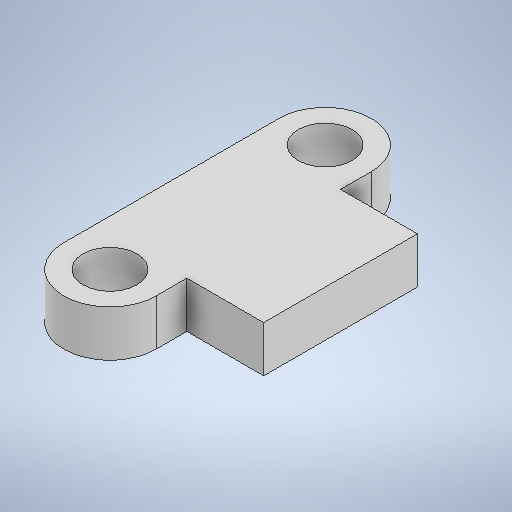
# Autodesk Inventor part: Top Bracket
Saved by Autodesk Inventor 2026.2 (Build 302298010, 298A)
## iProperties
Created: 2026-05-02
Part Number: Top Bracket
Material: Generic
Document SubType Name: Modeling
Designer: piete
Density: 1 g/cm^3
Appearance: Default
Author: piete
Autodesk Inventor part; units mm, degrees
ref_plane "YZ Plane" through (0, 0, 0) normal (1, 0, 0) x (0, 1, 0)
ref_plane "XZ Plane" through (0, 0, 0) normal (0, 1, 0) x (-1, 0, 0)
ref_plane "XY Plane" through (0, 0, 0) normal (0, 0, 1) x (1, 0, 0)
sketch "Sketch1" plane through (0, 0, 0) normal (0, 1, 0) x (-1, 0, 0)
  circle A0 centre (0, 7) radius 1.75
  circle A1 centre (0, -7) radius 1.75
  line L0 (3, 7) -> (-3, 7)
  line L1 (-3, 7) -> (-3, -7)
  line L2 (-3, -7) -> (3, -7)
  line L3 (3, -7) -> (3, 7)
  circle A2 centre (0, 7) radius 3
  circle A3 centre (0, -7) radius 3
  point P0 (0, 0)
  point P1 (-3, 7)
  dimension "d0" = 3.5
  dimension "d1" = 3.5
  dimension "d2" = 14
  dimension "d3" = 7
  dimension "d4" = 0
  dimension "d5" = 0
  dimension "d6" = 6
  dimension "d7" = 14
  dimension "d8" = 3
  dimension "d9" = 6
  dimension "d10" = 6
  dimension "d11" = 7
  constraints: 8 end point, 4 centre point, 2 coincident, 2 parallel, 1 horizontal, 1 perpendicular
  measures "d0" diameter of A0
  measures "d1" diameter of A1
  measures "d2" distance of A0.centre A1.centre
  measures "d3" distance of A0.centre point (0, 0)
  measures "d4" horizontal distance of point (0, 0) A1.centre
  measures "d5" horizontal distance of point (0, 0) A0.centre
  measures "d6" distance of L2.end L1.end
  measures "d7" distance of L1.end L0.end
  measures "d8" distance from line of L3 point (0, 0)
  measures "d9" diameter of A2
  measures "d10" diameter of A3
  measures "d11" distance from line of point (0, 0) L0
extrude "Extrusion1" add sketch "Sketch1" along normal blind 3 contours L0 A2 A0 | A0 L0 A2 | L3 A3 L1 A2 | A3 L2 A1 | L2 A1 A3
sketch "Sketch2" plane through (0, 3, 0) normal (0, 1, 0) x (1, 0, 0)
  line L0 (3, -7) -> (3, 7) projected
  line L1 (3, 5) -> (8, 5)
  line L2 (8, 5) -> (8, -5)
  line L3 (8, -5) -> (3, -5)
  line L4 (3, -5) -> (3, 5)
  point P0 (0, 0)
  dimension "d14" = 5
  dimension "d15" = 5
  dimension "d16" = 5
  constraints: 8 end point, 2 parallel, 1 horizontal, 1 perpendicular, 1 point on line
  measures "d14" distance of L2.end L3.end
  measures "d15" distance from line of point (0, 0) L1
  measures "d16" distance from line of point (0, 0) L3
extrude "Extrusion2" add sketch "Sketch2" against normal up to surface (3 mm away)
body "Solid1"
